Autodesk Inventor part; units mm, degrees
(part 2 of 4)
sketch "스케치25" plane through (0, 5, 0) normal (0, 1, 0) x (1, 0, 0)
  line L0 (49.6203, 83.501) -> (49.6203, 93.501) projected
  arc A0 (51.6203, 95.501) -> (49.6203, 93.501) centre (51.6203, 93.501) ccw projected
  line L1 (51.6203, 95.501) -> (90.0011, 95.501) projected
  arc A1 (92.0011, 93.501) -> (90.0011, 95.501) centre (90.0011, 93.501) ccw projected
  line L2 (92.0011, 93.501) -> (92.0011, 83.501) projected
  arc A2 (90.0011, 81.501) -> (92.0011, 83.501) centre (90.0011, 83.501) ccw projected
  line L3 (90.0011, 81.501) -> (51.6203, 81.501) projected
  arc A3 (49.6203, 83.501) -> (51.6203, 81.501) centre (51.6203, 83.501) ccw projected
  line L4 (127.7787, 126.9669) -> (13, 126.9669) projected
  line L5 (13, 126.9669) -> (-27.1, 106.9169) projected
  line L6 (-27.1, 106.9169) -> (-27.1, -28) projected
  line L7 (-27.1, -28) -> (27.1, -28) projected
  line L8 (27.1, -28) -> (27.1, 45.1435) projected
  arc A4 (28.3615, 47.0022) -> (27.1, 45.1435) centre (29.1, 45.1435) ccw projected
  line L9 (28.3615, 47.0022) -> (126.5171, 85.9998) projected
  arc A5 (126.5171, 85.9998) -> (127.7787, 87.8585) centre (125.7787, 87.8585) ccw projected
  line L10 (127.7787, 126.9669) -> (127.7787, 87.8585) projected
  line L11 (15, 93.501) -> (15, 83.501) projected
  arc A6 (13, 81.501) -> (15, 83.501) centre (13, 83.501) ccw projected
  line L12 (13, 81.501) -> (-13, 81.501) projected
  arc A7 (-15, 83.501) -> (-13, 81.501) centre (-13, 83.501) ccw projected
  line L13 (-15, 83.501) -> (-15, 93.501) projected
  arc A8 (-13, 95.501) -> (-15, 93.501) centre (-13, 93.501) ccw projected
  line L14 (-13, 95.501) -> (13, 95.501) projected
  arc A9 (15, 93.501) -> (13, 95.501) centre (13, 93.501) ccw projected
  circle A10 centre (39.1, 76.501) radius 1.6 projected
  circle A11 centre (49.8107, 76.501) radius 1.6 projected
  circle A12 centre (9.1, 76.501) radius 1.6 projected
  circle A13 centre (-10.9, 76.501) radius 1.6 projected
  circle A14 centre (69.8107, 76.501) radius 1.6 projected
  circle A15 centre (89.8107, 76.501) radius 1.6 projected
  circle A16 centre (12.0104, 4.9749) radius 3.1 projected
  circle A17 centre (4.9749, -12.0104) radius 3.1 projected
  circle A18 centre (-12.0104, -4.9749) radius 3.1 projected
  circle A19 centre (-4.9749, 12.0104) radius 3.1 projected
  circle A20 centre (0, 0) radius 8 projected
  circle A21 centre (-12.0104, 4.9749) radius 3.1 projected
  circle A22 centre (-4.9749, -12.0104) radius 3.1 projected
  circle A23 centre (12.0104, -4.9749) radius 3.1 projected
  circle A24 centre (4.9749, 12.0104) radius 3.1 projected
  circle A25 centre (70.8107, 118.101) radius 1.35 projected
  circle A26 centre (112.9107, 96.101) radius 1.75 projected
  circle A27 centre (58.8107, 106.101) radius 1.35 projected
  circle A28 centre (28.7107, 96.101) radius 1.75 projected
  circle A29 centre (82.8107, 106.101) radius 1.35 projected
  circle A30 centre (112.9107, 116.101) radius 1.75 projected
  circle A31 centre (28.7107, 116.101) radius 1.75 projected
  line L15 (49.6203, 85.501) -> (49.6203, 95.501)
  arc A32 (51.6203, 97.501) -> (49.6203, 95.501) centre (51.6203, 95.501) ccw
  line L16 (51.6203, 97.501) -> (90.0011, 97.501)
  arc A33 (92.0011, 95.501) -> (90.0011, 97.501) centre (90.0011, 95.501) ccw
  line L17 (92.0011, 95.501) -> (92.0011, 85.501)
  arc A34 (90.0011, 83.501) -> (92.0011, 85.501) centre (90.0011, 85.501) ccw
  line L18 (90.0011, 83.501) -> (51.6203, 83.501)
  arc A35 (49.6203, 85.501) -> (51.6203, 83.501) centre (51.6203, 85.501) ccw
  line L19 (127.7787, 128.9669) -> (13, 128.9669)
  line L20 (13, 128.9669) -> (-27.1, 108.9169)
  line L21 (-27.1, 108.9169) -> (-27.1, -26)
  line L22 (-27.1, -26) -> (27.1, -26)
  line L23 (27.1, -26) -> (27.1, 47.1435)
  arc A36 (28.3615, 49.0022) -> (27.1, 47.1435) centre (29.1, 47.1435) ccw
  line L24 (28.3615, 49.0022) -> (126.5171, 87.9998)
  arc A37 (126.5171, 87.9998) -> (127.7787, 89.8585) centre (125.7787, 89.8585) ccw
  line L25 (127.7787, 128.9669) -> (127.7787, 89.8585)
  line L26 (15, 95.501) -> (15, 85.501)
  arc A38 (13, 83.501) -> (15, 85.501) centre (13, 85.501) ccw
  line L27 (13, 83.501) -> (-13, 83.501)
  arc A39 (-15, 85.501) -> (-13, 83.501) centre (-13, 85.501) ccw
  line L28 (-15, 85.501) -> (-15, 95.501)
  arc A40 (-13, 97.501) -> (-15, 95.501) centre (-13, 95.501) ccw
  line L29 (-13, 97.501) -> (13, 97.501)
  arc A41 (15, 95.501) -> (13, 97.501) centre (13, 95.501) ccw
  circle A42 centre (39.1, 78.501) radius 1.6
  circle A43 centre (49.8107, 78.501) radius 1.6
  circle A44 centre (9.1, 78.501) radius 1.6
  circle A45 centre (-10.9, 78.501) radius 1.6
  circle A46 centre (69.8107, 78.501) radius 1.6
  circle A47 centre (89.8107, 78.501) radius 1.6
  circle A48 centre (12.0104, 6.9749) radius 3.1
  circle A49 centre (4.9749, -10.0104) radius 3.1
  circle A50 centre (-12.0104, -2.9749) radius 3.1
  circle A51 centre (-4.9749, 14.0104) radius 3.1
  circle A52 centre (0, 2) radius 8
  circle A53 centre (-12.0104, 6.9749) radius 3.1
  circle A54 centre (-4.9749, -10.0104) radius 3.1
  circle A55 centre (12.0104, -2.9749) radius 3.1
  circle A56 centre (4.9749, 14.0104) radius 3.1
  circle A57 centre (70.8107, 120.101) radius 1.35
  circle A58 centre (112.9107, 98.101) radius 1.75
  circle A59 centre (58.8107, 108.101) radius 1.35
  circle A60 centre (28.7107, 98.101) radius 1.75
  circle A61 centre (82.8107, 108.101) radius 1.35
  circle A62 centre (112.9107, 118.101) radius 1.75
  circle A63 centre (28.7107, 118.101) radius 1.75
  circle A64 centre (70.8107, 118.101) radius 1.35 projected
  line L30 (70.8107, 118.101) -> (70.8107, 120.101)
  point P0 (0, 2)
  dimension "d177" = 2
  constraints: 32 centre point, 32 end point, 20 point on circle, 1 vertical
  measures "d177" distance of L30.start L30.end
extrude "돌출28" add sketch "스케치25" against normal blind 5 contours A25 A57 | A57 L30 A25 | A25 L30 A57 | A26 A58 | A58 A26 | A27 A59 | A59 A27 | A28 A60 | A60 A28 | A29 A61 | A61 A29 | A30 A62 | A62 A30 | A31 A63 | A63 A31 picked at (70.7711, 117.4255) picked at (112.8481, 95.0285) picked at (112.7717, 97.3342) picked at (58.7711, 105.4255) picked at (58.9201, 106.9978) picked at (28.6481, 95.0285) picked at (28.5717, 97.3342) picked at (82.7711, 105.4255) picked at (82.7013, 106.9978) picked at (112.8481, 115.0285) picked at (112.7717, 117.3342) picked at (28.6481, 115.0285) picked at (28.5717, 117.3342)
extrude "돌출29" cut sketch "스케치25" against normal blind 5 contours A57 L30 A25 | A25 A57 | A25 L30 A57 | A58 A26 | A26 A58 | A59 A27 | A27 A59 | A60 A28 | A28 A60 | A61 A29 | A29 A61 | A62 A30 | A30 A62 | A63 A31 | A31 A63 picked at (70.7711, 120.7765) picked at (112.7717, 97.3342) picked at (112.8481, 99.1735) picked at (58.9201, 106.9978) picked at (58.7711, 108.7765) picked at (28.5717, 97.3342) picked at (28.6481, 99.1735) picked at (82.7013, 106.9978) picked at (82.7711, 108.7765) picked at (112.7717, 117.3342) picked at (112.8481, 119.1735) picked at (28.5717, 117.3342) picked at (28.6481, 119.1735)
fillet "모깎기4" radius 2 3 edges at (-27.1, 2.5, -106.9169) (13, 2.5, -126.9669) (127.7787, 2.5, -126.9669)
sketch "스케치26" plane through (0, 5, 0) normal (0, 1, 0) x (1, 0, 0)
  circle A0 centre (4.9749, 12.0104) radius 3.1 projected
  circle A1 centre (12.0104, -4.9749) radius 3.1 projected
  circle A2 centre (-4.9749, -12.0104) radius 3.1 projected
  circle A3 centre (-12.0104, 4.9749) radius 3.1 projected
  circle A4 centre (0, 0) radius 8 projected
  circle A5 centre (-4.9749, 12.0104) radius 3.1 projected
  circle A6 centre (-12.0104, -4.9749) radius 3.1 projected
  circle A7 centre (4.9749, -12.0104) radius 3.1 projected
  circle A8 centre (12.0104, 4.9749) radius 3.1 projected
  circle A9 centre (89.8107, 76.501) radius 1.6 projected
  circle A10 centre (69.8107, 76.501) radius 1.6 projected
  circle A11 centre (-10.9, 76.501) radius 1.6 projected
  circle A12 centre (9.1, 76.501) radius 1.6 projected
  circle A13 centre (49.8107, 76.501) radius 1.6 projected
  circle A14 centre (39.1, 76.501) radius 1.6 projected
  line L0 (15, 93.501) -> (15, 83.501) projected
  arc A15 (13, 81.501) -> (15, 83.501) centre (13, 83.501) ccw projected
  line L1 (13, 81.501) -> (-13, 81.501) projected
  arc A16 (-15, 83.501) -> (-13, 81.501) centre (-13, 83.501) ccw projected
  line L2 (-15, 83.501) -> (-15, 93.501) projected
  arc A17 (-13, 95.501) -> (-15, 93.501) centre (-13, 93.501) ccw projected
  line L3 (-13, 95.501) -> (13, 95.501) projected
  arc A18 (15, 93.501) -> (13, 95.501) centre (13, 93.501) ccw projected
  arc A19 (127.7787, 124.9669) -> (125.7787, 126.9669) centre (125.7787, 124.9669) ccw projected
  line L4 (125.7787, 126.9669) -> (13.4721, 126.9669) projected
  arc A20 (13.4721, 126.9669) -> (12.5777, 126.7557) centre (13.4721, 124.9669) ccw projected
  line L5 (12.5777, 126.7557) -> (-25.9944, 107.4697) projected
  arc A21 (-25.9944, 107.4697) -> (-27.1, 105.6808) centre (-25.1, 105.6808) ccw projected
  line L6 (-27.1, 105.6808) -> (-27.1, -28) projected
  line L7 (-27.1, -28) -> (27.1, -28) projected
  line L8 (27.1, -28) -> (27.1, 45.1435) projected
  arc A22 (28.3615, 47.0022) -> (27.1, 45.1435) centre (29.1, 45.1435) ccw projected
  line L9 (28.3615, 47.0022) -> (126.5171, 85.9998) projected
  arc A23 (126.5171, 85.9998) -> (127.7787, 87.8585) centre (125.7787, 87.8585) ccw projected
  line L10 (127.7787, 124.9669) -> (127.7787, 87.8585) projected
  line L11 (49.6203, 83.501) -> (49.6203, 93.501) projected
  arc A24 (51.6203, 95.501) -> (49.6203, 93.501) centre (51.6203, 93.501) ccw projected
  line L12 (51.6203, 95.501) -> (90.0011, 95.501) projected
  arc A25 (92.0011, 93.501) -> (90.0011, 95.501) centre (90.0011, 93.501) ccw projected
  line L13 (92.0011, 93.501) -> (92.0011, 83.501) projected
  arc A26 (90.0011, 81.501) -> (92.0011, 83.501) centre (90.0011, 83.501) ccw projected
  line L14 (90.0011, 81.501) -> (51.6203, 81.501) projected
  arc A27 (49.6203, 83.501) -> (51.6203, 81.501) centre (51.6203, 83.501) ccw projected
  circle A28 centre (28.7107, 98.101) radius 1.75 projected
  circle A29 centre (82.8107, 108.101) radius 1.35 projected
  circle A30 centre (112.9107, 118.101) radius 1.75 projected
  circle A31 centre (28.7107, 118.101) radius 1.75 projected
  circle A32 centre (70.8107, 120.101) radius 1.35 projected
  circle A33 centre (112.9107, 98.101) radius 1.75 projected
  circle A34 centre (58.8107, 108.101) radius 1.35 projected
  line L15 (-27.1, 105.6808) -> (-27.1, -28) projected
  line L16 (-27.1, 0) -> (27.1, 0)
  line L17 (27.1, -28) -> (27.1, 45.1435) projected
  point P0 (27.1, 0)
  constraints: 2 end point, 2 point on line
extrude "돌출30" cut sketch "스케치26" against normal blind 10 contours A1 | A2 | L16 L8 L7 L6 A4 | A4 L16 | A6 | A7 picked at (-2.3612, -1.2393)
sketch "스케치27" plane through (0, 5, 0) normal (0, 1, 0) x (1, 0, 0)
  circle A0 centre (58.8107, 108.101) radius 1.35 projected
  circle A1 centre (112.9107, 98.101) radius 1.75 projected
  circle A2 centre (70.8107, 120.101) radius 1.35 projected
  circle A3 centre (28.7107, 118.101) radius 1.75 projected
  circle A4 centre (112.9107, 118.101) radius 1.75 projected
  circle A5 centre (82.8107, 108.101) radius 1.35 projected
  circle A6 centre (28.7107, 98.101) radius 1.75 projected
  line L0 (49.6203, 83.501) -> (49.6203, 93.501) projected
  arc A7 (51.6203, 95.501) -> (49.6203, 93.501) centre (51.6203, 93.501) ccw projected
  line L1 (51.6203, 95.501) -> (90.0011, 95.501) projected
  arc A8 (92.0011, 93.501) -> (90.0011, 95.501) centre (90.0011, 93.501) ccw projected
  line L2 (92.0011, 93.501) -> (92.0011, 83.501) projected
  arc A9 (90.0011, 81.501) -> (92.0011, 83.501) centre (90.0011, 83.501) ccw projected
  line L3 (90.0011, 81.501) -> (51.6203, 81.501) projected
  arc A10 (49.6203, 83.501) -> (51.6203, 81.501) centre (51.6203, 83.501) ccw projected
  line L4 (-27.1, 0) -> (-8, 0) projected
  arc A11 (8, 0) -> (-8, 0) centre (0, 0) ccw projected
  line L5 (8, 0) -> (27.1, 0) projected
  line L6 (27.1, 0) -> (27.1, 45.1435) projected
  arc A12 (28.3615, 47.0022) -> (27.1, 45.1435) centre (29.1, 45.1435) ccw projected
  line L7 (28.3615, 47.0022) -> (126.5171, 85.9998) projected
  arc A13 (126.5171, 85.9998) -> (127.7787, 87.8585) centre (125.7787, 87.8585) ccw projected
  line L8 (127.7787, 124.9669) -> (127.7787, 87.8585) projected
  arc A14 (127.7787, 124.9669) -> (125.7787, 126.9669) centre (125.7787, 124.9669) ccw projected
  line L9 (125.7787, 126.9669) -> (13.4721, 126.9669) projected
  arc A15 (13.4721, 126.9669) -> (12.5777, 126.7557) centre (13.4721, 124.9669) ccw projected
  line L10 (12.5777, 126.7557) -> (-25.9944, 107.4697) projected
  arc A16 (-25.9944, 107.4697) -> (-27.1, 105.6808) centre (-25.1, 105.6808) ccw projected
  line L11 (-27.1, 105.6808) -> (-27.1, 0) projected
  line L12 (15, 93.501) -> (15, 83.501) projected
  arc A17 (13, 81.501) -> (15, 83.501) centre (13, 83.501) ccw projected
  line L13 (13, 81.501) -> (-13, 81.501) projected
  arc A18 (-15, 83.501) -> (-13, 81.501) centre (-13, 83.501) ccw projected
  line L14 (-15, 83.501) -> (-15, 93.501) projected
  arc A19 (-13, 95.501) -> (-15, 93.501) centre (-13, 93.501) ccw projected
  line L15 (-13, 95.501) -> (13, 95.501) projected
  arc A20 (15, 93.501) -> (13, 95.501) centre (13, 93.501) ccw projected
  circle A21 centre (39.1, 76.501) radius 1.6 projected
  circle A22 centre (49.8107, 76.501) radius 1.6 projected
  circle A23 centre (9.1, 76.501) radius 1.6 projected
  circle A24 centre (-10.9, 76.501) radius 1.6 projected
  circle A25 centre (69.8107, 76.501) radius 1.6 projected
  circle A26 centre (89.8107, 76.501) radius 1.6 projected
  circle A27 centre (12.0104, 4.9749) radius 3.1 projected
  circle A28 centre (-4.9749, 12.0104) radius 3.1 projected
  circle A29 centre (-12.0104, 4.9749) radius 3.1 projected
  circle A30 centre (4.9749, 12.0104) radius 3.1 projected
  circle A31 centre (12.0104, 4.9749) radius 1.6 projected
  circle A32 centre (4.9749, 12.0104) radius 1.6 projected
  circle A33 centre (-4.9749, 12.0104) radius 1.6 projected
  circle A34 centre (-12.0104, 4.9749) radius 1.6 projected
  line L16 (27.1, 0) -> (27.1, 45.1435) projected
  line L17 (-27.1, 0) -> (-27.1, 105.6808) projected
  line L18 (27.1, 0) -> (-27.1, 0)
  circle A35 centre (58.8107, -108.101) radius 1.35
  circle A36 centre (112.9107, -98.101) radius 1.75
  circle A37 centre (70.8107, -120.101) radius 1.35
  circle A38 centre (28.7107, -118.101) radius 1.75
  circle A39 centre (112.9107, -118.101) radius 1.75
  circle A40 centre (82.8107, -108.101) radius 1.35
  circle A41 centre (28.7107, -98.101) radius 1.75
  line L19 (49.6203, -83.501) -> (49.6203, -93.501)
  arc A42 (49.6203, -93.501) -> (51.6203, -95.501) centre (51.6203, -93.501) ccw
  line L20 (51.6203, -95.501) -> (90.0011, -95.501)
  arc A43 (90.0011, -95.501) -> (92.0011, -93.501) centre (90.0011, -93.501) ccw
  line L21 (92.0011, -93.501) -> (92.0011, -83.501)
  arc A44 (92.0011, -83.501) -> (90.0011, -81.501) centre (90.0011, -83.501) ccw
  line L22 (90.0011, -81.501) -> (51.6203, -81.501)
  arc A45 (51.6203, -81.501) -> (49.6203, -83.501) centre (51.6203, -83.501) ccw
  arc A46 (-8, 0) -> (8, 0) centre (0, 0) ccw
  line L23 (27.1, 0) -> (27.1, -45.1435)
  arc A47 (27.1, -45.1435) -> (28.3615, -47.0022) centre (29.1, -45.1435) ccw
  line L24 (28.3615, -47.0022) -> (126.5171, -85.9998)
  arc A48 (127.7787, -87.8585) -> (126.5171, -85.9998) centre (125.7787, -87.8585) ccw
  line L25 (127.7787, -124.9669) -> (127.7787, -87.8585)
  arc A49 (125.7787, -126.9669) -> (127.7787, -124.9669) centre (125.7787, -124.9669) ccw
  line L26 (125.7787, -126.9669) -> (13.4721, -126.9669)
  arc A50 (12.5777, -126.7557) -> (13.4721, -126.9669) centre (13.4721, -124.9669) ccw
  line L27 (12.5777, -126.7557) -> (-25.9944, -107.4697)
  arc A51 (-27.1, -105.6808) -> (-25.9944, -107.4697) centre (-25.1, -105.6808) ccw
  line L28 (-27.1, -105.6808) -> (-27.1, 0)
  line L29 (15, -93.501) -> (15, -83.501)
  arc A52 (15, -83.501) -> (13, -81.501) centre (13, -83.501) ccw
  line L30 (13, -81.501) -> (-13, -81.501)
  arc A53 (-13, -81.501) -> (-15, -83.501) centre (-13, -83.501) ccw
  line L31 (-15, -83.501) -> (-15, -93.501)
  arc A54 (-15, -93.501) -> (-13, -95.501) centre (-13, -93.501) ccw
  line L32 (-13, -95.501) -> (13, -95.501)
  arc A55 (13, -95.501) -> (15, -93.501) centre (13, -93.501) ccw
  circle A56 centre (39.1, -76.501) radius 1.6
  circle A57 centre (49.8107, -76.501) radius 1.6
  circle A58 centre (9.1, -76.501) radius 1.6
  circle A59 centre (-10.9, -76.501) radius 1.6
  circle A60 centre (69.8107, -76.501) radius 1.6
  circle A61 centre (89.8107, -76.501) radius 1.6
  circle A62 centre (12.0104, -4.9749) radius 3.1
  circle A63 centre (-4.9749, -12.0104) radius 3.1
  circle A64 centre (-12.0104, -4.9749) radius 3.1
  circle A65 centre (4.9749, -12.0104) radius 3.1
  circle A66 centre (12.0104, -4.9749) radius 1.6
  circle A67 centre (4.9749, -12.0104) radius 1.6
  circle A68 centre (-4.9749, -12.0104) radius 1.6
  circle A69 centre (-12.0104, -4.9749) radius 1.6
  line L33 (27.1, 0) -> (27.1, -45.1435)
  line L34 (-27.1, 0) -> (-27.1, -105.6808)
  constraints: 60 symmetric about line, 35 centre point, 34 end point, 28 point on circle, 1 perpendicular, 35 other
extrude "돌출31" add sketch "스케치27" against normal blind 5 contours L4 A46 L5 L23 A47 L24 A48 L25 A49 L26 A50 L27 A51 L28
sketch "스케치28" plane through (0, 5, 0) normal (0, 1, 0) x (1, 0, 0)
  line L0 (27.1, -45.1435) -> (27.1, 45.1435) projected
  arc A0 (28.3615, 47.0022) -> (27.1, 45.1435) centre (29.1, 45.1435) ccw projected
  line L1 (28.3615, 47.0022) -> (126.5171, 85.9998) projected
  arc A1 (126.5171, 85.9998) -> (127.7787, 87.8585) centre (125.7787, 87.8585) ccw projected
  line L2 (127.7787, 124.9669) -> (127.7787, 87.8585) projected
  arc A2 (127.7787, 124.9669) -> (125.7787, 126.9669) centre (125.7787, 124.9669) ccw projected
  line L3 (125.7787, 126.9669) -> (13.4721, 126.9669) projected
  arc A3 (13.4721, 126.9669) -> (12.5777, 126.7557) centre (13.4721, 124.9669) ccw projected
  line L4 (12.5777, 126.7557) -> (-25.9944, 107.4697) projected
  arc A4 (-25.9944, 107.4697) -> (-27.1, 105.6808) centre (-25.1, 105.6808) ccw projected
  line L5 (-27.1, 105.6808) -> (-27.1, -105.6808) projected
  arc A5 (-27.1, -105.6808) -> (-25.9944, -107.4697) centre (-25.1, -105.6808) ccw projected
  line L6 (-25.9944, -107.4697) -> (12.5777, -126.7557) projected
  arc A6 (12.5777, -126.7557) -> (13.4721, -126.9669) centre (13.4721, -124.9669) ccw projected
  line L7 (13.4721, -126.9669) -> (125.7787, -126.9669) projected
  arc A7 (125.7787, -126.9669) -> (127.7787, -124.9669) centre (125.7787, -124.9669) ccw projected
  line L8 (127.7787, -124.9669) -> (127.7787, -87.8585) projected
  arc A8 (127.7787, -87.8585) -> (126.5171, -85.9998) centre (125.7787, -87.8585) ccw projected
  line L9 (126.5171, -85.9998) -> (28.3615, -47.0022) projected
  arc A9 (27.1, -45.1435) -> (28.3615, -47.0022) centre (29.1, -45.1435) ccw projected
  arc A10 (15, -83.501) -> (13, -81.501) centre (13, -83.501) ccw projected
  line L10 (15, -83.501) -> (15, -93.501) projected
  arc A11 (13, -95.501) -> (15, -93.501) centre (13, -93.501) ccw projected
  line L11 (13, -95.501) -> (-13, -95.501) projected
  arc A12 (-15, -93.501) -> (-13, -95.501) centre (-13, -93.501) ccw projected
  line L12 (-15, -93.501) -> (-15, -83.501) projected
  arc A13 (-13, -81.501) -> (-15, -83.501) centre (-13, -83.501) ccw projected
  line L13 (-13, -81.501) -> (13, -81.501) projected
  line L14 (49.6203, -93.501) -> (49.6203, -83.501) projected
  arc A14 (51.6203, -81.501) -> (49.6203, -83.501) centre (51.6203, -83.501) ccw projected
  line L15 (51.6203, -81.501) -> (90.0011, -81.501) projected
  arc A15 (92.0011, -83.501) -> (90.0011, -81.501) centre (90.0011, -83.501) ccw projected
  line L16 (92.0011, -83.501) -> (92.0011, -93.501) projected
  arc A16 (90.0011, -95.501) -> (92.0011, -93.501) centre (90.0011, -93.501) ccw projected
  line L17 (90.0011, -95.501) -> (51.6203, -95.501) projected
  arc A17 (49.6203, -93.501) -> (51.6203, -95.501) centre (51.6203, -93.501) ccw projected
  circle A18 centre (49.8107, -76.501) radius 1.6 projected
  circle A19 centre (39.1, -76.501) radius 1.6 projected
  circle A20 centre (69.8107, -76.501) radius 1.6 projected
  circle A21 centre (89.8107, -76.501) radius 1.6 projected
  circle A22 centre (-4.9749, -12.0104) radius 3.1 projected
  circle A23 centre (4.9749, -12.0104) radius 3.1 projected
  circle A24 centre (-12.0104, -4.9749) radius 3.1 projected
  circle A25 centre (12.0104, -4.9749) radius 3.1 projected
  circle A26 centre (9.1, -76.501) radius 1.6 projected
  circle A27 centre (112.9107, -98.101) radius 1.75 projected
  circle A28 centre (82.8107, -108.101) radius 1.35 projected
  circle A29 centre (58.8107, -108.101) radius 1.35 projected
  circle A30 centre (28.7107, -118.101) radius 1.75 projected
  circle A31 centre (28.7107, -98.101) radius 1.75 projected
  circle A32 centre (70.8107, -120.101) radius 1.35 projected
  circle A33 centre (112.9107, -118.101) radius 1.75 projected
  circle A34 centre (-10.9, -76.501) radius 1.6 projected
  circle A35 centre (58.8107, 108.101) radius 1.35 projected
  circle A36 centre (112.9107, 98.101) radius 1.75 projected
  circle A37 centre (70.8107, 120.101) radius 1.35 projected
  circle A38 centre (28.7107, 118.101) radius 1.75 projected
  circle A39 centre (112.9107, 118.101) radius 1.75 projected
  circle A40 centre (82.8107, 108.101) radius 1.35 projected
  circle A41 centre (28.7107, 98.101) radius 1.75 projected
  line L18 (49.6203, 83.501) -> (49.6203, 93.501) projected
  arc A42 (51.6203, 95.501) -> (49.6203, 93.501) centre (51.6203, 93.501) ccw projected
  line L19 (51.6203, 95.501) -> (90.0011, 95.501) projected
  arc A43 (92.0011, 93.501) -> (90.0011, 95.501) centre (90.0011, 93.501) ccw projected
  line L20 (92.0011, 93.501) -> (92.0011, 83.501) projected
  arc A44 (90.0011, 81.501) -> (92.0011, 83.501) centre (90.0011, 83.501) ccw projected
  line L21 (90.0011, 81.501) -> (51.6203, 81.501) projected
  arc A45 (49.6203, 83.501) -> (51.6203, 81.501) centre (51.6203, 83.501) ccw projected
  circle A46 centre (0, 0) radius 8 projected
  line L22 (15, 93.501) -> (15, 83.501) projected
  arc A47 (13, 81.501) -> (15, 83.501) centre (13, 83.501) ccw projected
  line L23 (13, 81.501) -> (-13, 81.501) projected
  arc A48 (-15, 83.501) -> (-13, 81.501) centre (-13, 83.501) ccw projected
  line L24 (-15, 83.501) -> (-15, 93.501) projected
  arc A49 (-13, 95.501) -> (-15, 93.501) centre (-13, 93.501) ccw projected
  line L25 (-13, 95.501) -> (13, 95.501) projected
  arc A50 (15, 93.501) -> (13, 95.501) centre (13, 93.501) ccw projected
  circle A51 centre (39.1, 76.501) radius 1.6 projected
  circle A52 centre (49.8107, 76.501) radius 1.6 projected
  circle A53 centre (9.1, 76.501) radius 1.6 projected
  circle A54 centre (-10.9, 76.501) radius 1.6 projected
  circle A55 centre (69.8107, 76.501) radius 1.6 projected
  circle A56 centre (89.8107, 76.501) radius 1.6 projected
  circle A57 centre (12.0104, 4.9749) radius 3.1 projected
  circle A58 centre (-4.9749, 12.0104) radius 3.1 projected
  circle A59 centre (-12.0104, 4.9749) radius 3.1 projected
  circle A60 centre (4.9749, 12.0104) radius 3.1 projected
  circle A61 centre (28.7107, 118.101) radius 1.75 projected
  line L26 (28.7107, 98.101) -> (28.7107, 118.101)
  circle A62 centre (35.7787, 108.101) radius 1.75
  circle A63 centre (15.7787, 108.101) radius 1.85
  line L27 (27.1, -45.1435) -> (27.1, 45.1435) projected
  line L28 (27.1, 0) -> (-27.1, 0)
  line L29 (-27.1, -105.6808) -> (-27.1, 105.6808) projected
  line L30 (125.7787, -126.9669) -> (13.4721, -126.9669)
  circle A64 centre (28.7107, -118.101) radius 1.75
  circle A65 centre (28.7107, -98.101) radius 1.75
  circle A66 centre (28.7107, -118.101) radius 1.75
  line L31 (28.7107, -98.101) -> (28.7107, -118.101)
  circle A67 centre (25.7787, -108.5308) radius 10.0092
  circle A68 centre (35.7787, -108.101) radius 1.75
  circle A69 centre (15.7787, -108.101) radius 1.85
  circle A70 centre (112.9107, 118.101) radius 1.75
  circle A71 centre (109.9787, 98.101) radius 1.75
  circle A72 centre (109.9787, 118.101) radius 1.75
  line L32 (109.9787, 98.101) -> (109.9787, 118.101)
  circle A73 centre (119.9787, 108.101) radius 1.75
  circle A74 centre (99.9787, 108.101) radius 1.85
  circle A75 centre (112.9107, 118.101) radius 1.75 projected
  line L33 (112.9107, 118.101) -> (112.9107, 98.101)
  circle A76 centre (112.9107, -98.101) radius 1.75
  circle A77 centre (112.9107, -118.101) radius 1.75
  circle A78 centre (112.9107, -118.101) radius 1.75
  circle A79 centre (119.9787, -108.101) radius 1.75
  circle A80 centre (109.9787, -98.101) radius 1.75
  line L34 (109.9787, -98.101) -> (109.9787, -118.101)
  circle A81 centre (109.9787, -118.101) radius 1.75
  circle A82 centre (109.9787, -108.101) radius 10
  circle A83 centre (99.9787, -108.101) radius 1.85
  circle A84 centre (112.9107, -118.101) radius 1.75
  line L35 (112.9107, -118.101) -> (112.9107, -98.101)
  point P0 (112.9107, 108.101)
  point P1 (112.9107, -108.101)
  dimension "d187" = 3.5
  dimension "d188" = 3.7
  dimension "d191" = 3.5
  dimension "d192" = 3.7
  dimension "d196" = 20
  dimension "d197" = 18.8659
  dimension "d198" = 7.8
  dimension "d199" = 64.2
  dimension "d200" = 20
  constraints: 22 centre point, 14 end point, 14 symmetric about line, 6 point on circle, 3 midpoint, 3 vertical, 16 other
  measures "d187" diameter of A62
  measures "d188" diameter of A63
  measures "d191" diameter of A73
  measures "d192" diameter of A74
  measures "d196" distance of A74.centre A73.centre
  measures "d197" distance from line of L3 A73.centre
  measures "d198" distance from line of L2 A73.centre
  measures "d199" distance of A62.centre A74.centre
  measures "d200" distance of A63.centre A62.centre
extrude "돌출32" cut sketch "스케치28" against normal blind 5 contours A82 A79 | A79 A82 | A83 A82 | A82 A83 | A68 A67 | A67 A68 | A69 A67 | A67 A69 | A62 | A63 | A73 | A74
sketch "스케치29" plane through (0, 5, 0) normal (0, 1, 0) x (1, 0, 0)
  circle A0 centre (99.9787, 108.101) radius 1.85 projected
  circle A1 centre (15.7787, -108.101) radius 1.85 projected
  circle A2 centre (35.7787, 108.101) radius 1.75 projected
  circle A3 centre (119.9787, -108.101) radius 1.75 projected
  circle A4 centre (119.9787, 108.101) radius 1.75 projected
  circle A5 centre (35.7787, -108.101) radius 1.75 projected
  circle A6 centre (15.7787, 108.101) radius 1.85 projected
  circle A7 centre (99.9787, -108.101) radius 1.85 projected
  line L0 (27.1, -45.1435) -> (27.1, 45.1435) projected
  arc A8 (28.3615, 47.0022) -> (27.1, 45.1435) centre (29.1, 45.1435) ccw projected
  line L1 (28.3615, 47.0022) -> (126.5171, 85.9998) projected
  arc A9 (126.5171, 85.9998) -> (127.7787, 87.8585) centre (125.7787, 87.8585) ccw projected
  line L2 (127.7787, 124.9669) -> (127.7787, 87.8585) projected
  arc A10 (127.7787, 124.9669) -> (125.7787, 126.9669) centre (125.7787, 124.9669) ccw projected
  line L3 (125.7787, 126.9669) -> (13.4721, 126.9669) projected
  arc A11 (13.4721, 126.9669) -> (12.5777, 126.7557) centre (13.4721, 124.9669) ccw projected
  line L4 (12.5777, 126.7557) -> (-25.9944, 107.4697) projected
  arc A12 (-25.9944, 107.4697) -> (-27.1, 105.6808) centre (-25.1, 105.6808) ccw projected
  line L5 (-27.1, 105.6808) -> (-27.1, -105.6808) projected
  arc A13 (-27.1, -105.6808) -> (-25.9944, -107.4697) centre (-25.1, -105.6808) ccw projected
  line L6 (-25.9944, -107.4697) -> (12.5777, -126.7557) projected
  arc A14 (12.5777, -126.7557) -> (13.4721, -126.9669) centre (13.4721, -124.9669) ccw projected
  line L7 (13.4721, -126.9669) -> (125.7787, -126.9669) projected
  arc A15 (125.7787, -126.9669) -> (127.7787, -124.9669) centre (125.7787, -124.9669) ccw projected
  line L8 (127.7787, -124.9669) -> (127.7787, -87.8585) projected
  arc A16 (127.7787, -87.8585) -> (126.5171, -85.9998) centre (125.7787, -87.8585) ccw projected
  line L9 (126.5171, -85.9998) -> (28.3615, -47.0022) projected
  arc A17 (27.1, -45.1435) -> (28.3615, -47.0022) centre (29.1, -45.1435) ccw projected
  arc A18 (15, -83.501) -> (13, -81.501) centre (13, -83.501) ccw projected
  line L10 (15, -83.501) -> (15, -93.501) projected
  arc A19 (13, -95.501) -> (15, -93.501) centre (13, -93.501) ccw projected
  line L11 (13, -95.501) -> (-13, -95.501) projected
  arc A20 (-15, -93.501) -> (-13, -95.501) centre (-13, -93.501) ccw projected
  line L12 (-15, -93.501) -> (-15, -83.501) projected
  arc A21 (-13, -81.501) -> (-15, -83.501) centre (-13, -83.501) ccw projected
  line L13 (-13, -81.501) -> (13, -81.501) projected
  line L14 (49.6203, -93.501) -> (49.6203, -83.501) projected
  arc A22 (51.6203, -81.501) -> (49.6203, -83.501) centre (51.6203, -83.501) ccw projected
  line L15 (51.6203, -81.501) -> (90.0011, -81.501) projected
  arc A23 (92.0011, -83.501) -> (90.0011, -81.501) centre (90.0011, -83.501) ccw projected
  line L16 (92.0011, -83.501) -> (92.0011, -93.501) projected
  arc A24 (90.0011, -95.501) -> (92.0011, -93.501) centre (90.0011, -93.501) ccw projected
  line L17 (90.0011, -95.501) -> (51.6203, -95.501) projected
  arc A25 (49.6203, -93.501) -> (51.6203, -95.501) centre (51.6203, -93.501) ccw projected
  circle A26 centre (49.8107, -76.501) radius 1.6 projected
  circle A27 centre (39.1, -76.501) radius 1.6 projected
  circle A28 centre (69.8107, -76.501) radius 1.6 projected
  circle A29 centre (89.8107, -76.501) radius 1.6 projected
  circle A30 centre (-4.9749, -12.0104) radius 3.1 projected
  circle A31 centre (4.9749, -12.0104) radius 3.1 projected
  circle A32 centre (-12.0104, -4.9749) radius 3.1 projected
  circle A33 centre (12.0104, -4.9749) radius 3.1 projected
  circle A34 centre (9.1, -76.501) radius 1.6 projected
  circle A35 centre (112.9107, -98.101) radius 1.75 projected
  circle A36 centre (82.8107, -108.101) radius 1.35 projected
  circle A37 centre (58.8107, -108.101) radius 1.35 projected
  circle A38 centre (28.7107, -118.101) radius 1.75 projected
  circle A39 centre (28.7107, -98.101) radius 1.75 projected
  circle A40 centre (70.8107, -120.101) radius 1.35 projected
  circle A41 centre (112.9107, -118.101) radius 1.75 projected
  circle A42 centre (-10.9, -76.501) radius 1.6 projected
  circle A43 centre (58.8107, 108.101) radius 1.35 projected
  circle A44 centre (112.9107, 98.101) radius 1.75 projected
  circle A45 centre (70.8107, 120.101) radius 1.35 projected
  circle A46 centre (28.7107, 118.101) radius 1.75 projected
  circle A47 centre (112.9107, 118.101) radius 1.75 projected
  circle A48 centre (82.8107, 108.101) radius 1.35 projected
  circle A49 centre (28.7107, 98.101) radius 1.75 projected
  line L18 (49.6203, 83.501) -> (49.6203, 93.501) projected
  arc A50 (51.6203, 95.501) -> (49.6203, 93.501) centre (51.6203, 93.501) ccw projected
  line L19 (51.6203, 95.501) -> (90.0011, 95.501) projected
  arc A51 (92.0011, 93.501) -> (90.0011, 95.501) centre (90.0011, 93.501) ccw projected
  line L20 (92.0011, 93.501) -> (92.0011, 83.501) projected
  arc A52 (90.0011, 81.501) -> (92.0011, 83.501) centre (90.0011, 83.501) ccw projected
  line L21 (90.0011, 81.501) -> (51.6203, 81.501) projected
  arc A53 (49.6203, 83.501) -> (51.6203, 81.501) centre (51.6203, 83.501) ccw projected
  circle A54 centre (0, 0) radius 8 projected
  line L22 (15, 93.501) -> (15, 83.501) projected
  arc A55 (13, 81.501) -> (15, 83.501) centre (13, 83.501) ccw projected
  line L23 (13, 81.501) -> (-13, 81.501) projected
  arc A56 (-15, 83.501) -> (-13, 81.501) centre (-13, 83.501) ccw projected
  line L24 (-15, 83.501) -> (-15, 93.501) projected
  arc A57 (-13, 95.501) -> (-15, 93.501) centre (-13, 93.501) ccw projected
  line L25 (-13, 95.501) -> (13, 95.501) projected
  arc A58 (15, 93.501) -> (13, 95.501) centre (13, 93.501) ccw projected
  circle A59 centre (39.1, 76.501) radius 1.6 projected
  circle A60 centre (49.8107, 76.501) radius 1.6 projected
  circle A61 centre (9.1, 76.501) radius 1.6 projected
  circle A62 centre (-10.9, 76.501) radius 1.6 projected
  circle A63 centre (69.8107, 76.501) radius 1.6 projected
  circle A64 centre (89.8107, 76.501) radius 1.6 projected
  circle A65 centre (12.0104, 4.9749) radius 3.1 projected
  circle A66 centre (-4.9749, 12.0104) radius 3.1 projected
  circle A67 centre (-12.0104, 4.9749) radius 3.1 projected
  circle A68 centre (4.9749, 12.0104) radius 3.1 projected
  arc A69 (28.3615, 47.0022) -> (27.1, 45.1435) centre (29.1, 45.1435) ccw projected
  line L26 (27.1, 45.1435) -> (27.1, 33.1435)
  line L27 (27.1, 33.1435) -> (127.7787, 73.1435)
  line L28 (28.3615, 47.0022) -> (126.5171, 85.9998) projected
  arc A70 (126.5171, 85.9998) -> (127.7787, 87.8585) centre (125.7787, 87.8585) ccw projected
  line L29 (127.7787, 87.8585) -> (127.7787, 73.1435)
  line L30 (27.1, -45.1435) -> (27.1, 45.1435) projected
  line L31 (27.1, 0) -> (-27.1, 0)
  line L32 (-27.1, 105.6808) -> (-27.1, -105.6808) projected
  line L33 (27.1, -33.1435) -> (127.7787, -73.1435)
  line L34 (127.7787, -87.8585) -> (127.7787, -73.1435)
  arc A71 (-25.9944, 107.4697) -> (-27.1, 105.6808) centre (-25.1, 105.6808) ccw projected
  line L35 (-27.1, 105.6808) -> (-27.1, 132.9669)
  arc A72 (127.7787, 124.9669) -> (125.7787, 126.9669) centre (125.7787, 124.9669) ccw projected
  line L36 (127.7787, 124.9669) -> (127.7787, 132.9669)
  line L37 (127.7787, 132.9669) -> (-27.1, 132.9669)
  line L38 (-27.1, -105.6808) -> (-27.1, -132.9669)
  line L39 (127.7787, -124.9669) -> (127.7787, -132.9669)
  line L40 (127.7787, -132.9669) -> (-27.1, -132.9669)
  point P0 (27.1, -33.1435)
  dimension "d201" = 12
  dimension "d204" = 8
  constraints: 24 end point, 4 symmetric about line, 3 tangent, 3 vertical, 2 midpoint, 1 parallel, 1 perpendicular, 1 point on line
  measures "d201" distance of L0.end L26.end
  measures "d204" distance of L2.start L36.end
extrude "돌출33" add sketch "스케치29" against normal blind 5 contours L0 L33 L34 A16 L9 A17 | L0 A8 L1 A9 L29 L27 | L39 L40 L38 A13 L6 A14 L7 A15 | A10 L3 A11 L4 A12 L35 L37 L36
fillet "모깎기5" radius 12 8 edges at (127.7787, 2.5, -132.9669) (127.7787, 2.5, -73.1435) (27.1, 2.5, -33.1435) (27.1, 2.5, 33.1435) (127.7787, 2.5, 73.1435) (127.7787, 2.5, 132.9669) (-27.1, 2.5, 132.9669) (-27.1, 2.5, -132.9669)
sketch "스케치30" plane through (0, 5, 0) normal (0, 1, 0) x (1, 0, 0)
  circle A0 centre (99.9787, 108.101) radius 1.85 projected
  circle A1 centre (15.7787, -108.101) radius 1.85 projected
  circle A2 centre (35.7787, 108.101) radius 1.75 projected
  circle A3 centre (119.9787, -108.101) radius 1.75 projected
  circle A4 centre (119.9787, 108.101) radius 1.75 projected
  circle A5 centre (35.7787, -108.101) radius 1.75 projected
  circle A6 centre (15.7787, 108.101) radius 1.85 projected
  circle A7 centre (99.9787, -108.101) radius 1.85 projected
  arc A8 (-15.1, 132.9669) -> (-27.1, 120.9669) centre (-15.1, 120.9669) ccw projected
  line L0 (-27.1, 120.9669) -> (-27.1, -120.9669) projected
  arc A9 (-27.1, -120.9669) -> (-15.1, -132.9669) centre (-15.1, -120.9669) ccw projected
  line L1 (-15.1, -132.9669) -> (115.7787, -132.9669) projected
  arc A10 (115.7787, -132.9669) -> (127.7787, -120.9669) centre (115.7787, -120.9669) ccw projected
  line L2 (127.7787, -120.9669) -> (127.7787, -81.2883) projected
  arc A11 (127.7787, -81.2883) -> (120.2094, -70.1362) centre (115.7787, -81.2883) ccw projected
  line L3 (120.2094, -70.1362) -> (34.6692, -36.1508) projected
  arc A12 (27.1, -24.9988) -> (34.6692, -36.1508) centre (39.1, -24.9988) ccw projected
  line L4 (27.1, -24.9988) -> (27.1, 24.9988) projected
  arc A13 (34.6692, 36.1508) -> (27.1, 24.9988) centre (39.1, 24.9988) ccw projected
  line L5 (34.6692, 36.1508) -> (120.2094, 70.1362) projected
  arc A14 (120.2094, 70.1362) -> (127.7787, 81.2883) centre (115.7787, 81.2883) ccw projected
  line L6 (127.7787, 81.2883) -> (127.7787, 120.9669) projected
  arc A15 (127.7787, 120.9669) -> (115.7787, 132.9669) centre (115.7787, 120.9669) ccw projected
  line L7 (115.7787, 132.9669) -> (-15.1, 132.9669) projected
  arc A16 (15, -83.501) -> (13, -81.501) centre (13, -83.501) ccw projected
  line L8 (15, -83.501) -> (15, -93.501) projected
  arc A17 (13, -95.501) -> (15, -93.501) centre (13, -93.501) ccw projected
  line L9 (13, -95.501) -> (-13, -95.501) projected
  arc A18 (-15, -93.501) -> (-13, -95.501) centre (-13, -93.501) ccw projected
  line L10 (-15, -93.501) -> (-15, -83.501) projected
  arc A19 (-13, -81.501) -> (-15, -83.501) centre (-13, -83.501) ccw projected
  line L11 (-13, -81.501) -> (13, -81.501) projected
  line L12 (49.6203, -93.501) -> (49.6203, -83.501) projected
  arc A20 (51.6203, -81.501) -> (49.6203, -83.501) centre (51.6203, -83.501) ccw projected
  line L13 (51.6203, -81.501) -> (90.0011, -81.501) projected
  arc A21 (92.0011, -83.501) -> (90.0011, -81.501) centre (90.0011, -83.501) ccw projected
  line L14 (92.0011, -83.501) -> (92.0011, -93.501) projected
  arc A22 (90.0011, -95.501) -> (92.0011, -93.501) centre (90.0011, -93.501) ccw projected
  line L15 (90.0011, -95.501) -> (51.6203, -95.501) projected
  arc A23 (49.6203, -93.501) -> (51.6203, -95.501) centre (51.6203, -93.501) ccw projected
  circle A24 centre (49.8107, -76.501) radius 1.6 projected
  circle A25 centre (39.1, -76.501) radius 1.6 projected
  circle A26 centre (69.8107, -76.501) radius 1.6 projected
  circle A27 centre (89.8107, -76.501) radius 1.6 projected
  circle A28 centre (-4.9749, -12.0104) radius 3.1 projected
  circle A29 centre (4.9749, -12.0104) radius 3.1 projected
  circle A30 centre (-12.0104, -4.9749) radius 3.1 projected
  circle A31 centre (12.0104, -4.9749) radius 3.1 projected
  circle A32 centre (9.1, -76.501) radius 1.6 projected
  circle A33 centre (112.9107, -98.101) radius 1.75 projected
  circle A34 centre (82.8107, -108.101) radius 1.35 projected
  circle A35 centre (58.8107, -108.101) radius 1.35 projected
  circle A36 centre (28.7107, -118.101) radius 1.75 projected
  circle A37 centre (28.7107, -98.101) radius 1.75 projected
  circle A38 centre (70.8107, -120.101) radius 1.35 projected
  circle A39 centre (112.9107, -118.101) radius 1.75 projected
  circle A40 centre (-10.9, -76.501) radius 1.6 projected
  circle A41 centre (58.8107, 108.101) radius 1.35 projected
  circle A42 centre (112.9107, 98.101) radius 1.75 projected
  circle A43 centre (70.8107, 120.101) radius 1.35 projected
  circle A44 centre (28.7107, 118.101) radius 1.75 projected
  circle A45 centre (112.9107, 118.101) radius 1.75 projected
  circle A46 centre (82.8107, 108.101) radius 1.35 projected
  circle A47 centre (28.7107, 98.101) radius 1.75 projected
  line L16 (49.6203, 83.501) -> (49.6203, 93.501) projected
  arc A48 (51.6203, 95.501) -> (49.6203, 93.501) centre (51.6203, 93.501) ccw projected
  line L17 (51.6203, 95.501) -> (90.0011, 95.501) projected
  arc A49 (92.0011, 93.501) -> (90.0011, 95.501) centre (90.0011, 93.501) ccw projected
  line L18 (92.0011, 93.501) -> (92.0011, 83.501) projected
  arc A50 (90.0011, 81.501) -> (92.0011, 83.501) centre (90.0011, 83.501) ccw projected
  line L19 (90.0011, 81.501) -> (51.6203, 81.501) projected
  arc A51 (49.6203, 83.501) -> (51.6203, 81.501) centre (51.6203, 83.501) ccw projected
  circle A52 centre (0, 0) radius 8 projected
  line L20 (15, 93.501) -> (15, 83.501) projected
  arc A53 (13, 81.501) -> (15, 83.501) centre (13, 83.501) ccw projected
  line L21 (13, 81.501) -> (-13, 81.501) projected
  arc A54 (-15, 83.501) -> (-13, 81.501) centre (-13, 83.501) ccw projected
  line L22 (-15, 83.501) -> (-15, 93.501) projected
  arc A55 (-13, 95.501) -> (-15, 93.501) centre (-13, 93.501) ccw projected
  line L23 (-13, 95.501) -> (13, 95.501) projected
  arc A56 (15, 93.501) -> (13, 95.501) centre (13, 93.501) ccw projected
  circle A57 centre (39.1, 76.501) radius 1.6 projected
  circle A58 centre (49.8107, 76.501) radius 1.6 projected
  circle A59 centre (9.1, 76.501) radius 1.6 projected
  circle A60 centre (-10.9, 76.501) radius 1.6 projected
  circle A61 centre (69.8107, 76.501) radius 1.6 projected
  circle A62 centre (89.8107, 76.501) radius 1.6 projected
  circle A63 centre (12.0104, 4.9749) radius 3.1 projected
  circle A64 centre (-4.9749, 12.0104) radius 3.1 projected
  circle A65 centre (-12.0104, 4.9749) radius 3.1 projected
  circle A66 centre (4.9749, 12.0104) radius 3.1 projected
extrude "돌출34" add sketch "스케치30" against normal blind 5 contours A33 | A34 | A35 | A36 | A37 | A38 | A39 | A41 | A42 | A43 | A44 | A45 | A46 | A47
sketch "스케치31" plane through (0, 5, 0) normal (0, 1, 0) x (1, 0, 0)
  circle A0 centre (99.9787, 108.101) radius 1.85 projected
  circle A1 centre (15.7787, -108.101) radius 1.85 projected
  circle A2 centre (35.7787, 108.101) radius 1.75 projected
  circle A3 centre (119.9787, -108.101) radius 1.75 projected
  circle A4 centre (119.9787, 108.101) radius 1.75 projected
  circle A5 centre (35.7787, -108.101) radius 1.75 projected
  circle A6 centre (15.7787, 108.101) radius 1.85 projected
  circle A7 centre (99.9787, -108.101) radius 1.85 projected
  arc A8 (-15.1, 132.9669) -> (-27.1, 120.9669) centre (-15.1, 120.9669) ccw projected
  line L0 (-27.1, 120.9669) -> (-27.1, -120.9669) projected
  arc A9 (-27.1, -120.9669) -> (-15.1, -132.9669) centre (-15.1, -120.9669) ccw projected
  line L1 (-15.1, -132.9669) -> (115.7787, -132.9669) projected
  arc A10 (115.7787, -132.9669) -> (127.7787, -120.9669) centre (115.7787, -120.9669) ccw projected
  line L2 (127.7787, -120.9669) -> (127.7787, -81.2883) projected
  arc A11 (127.7787, -81.2883) -> (120.2094, -70.1362) centre (115.7787, -81.2883) ccw projected
  line L3 (120.2094, -70.1362) -> (34.6692, -36.1508) projected
  arc A12 (27.1, -24.9988) -> (34.6692, -36.1508) centre (39.1, -24.9988) ccw projected
  line L4 (27.1, -24.9988) -> (27.1, 24.9988) projected
  arc A13 (34.6692, 36.1508) -> (27.1, 24.9988) centre (39.1, 24.9988) ccw projected
  line L5 (34.6692, 36.1508) -> (120.2094, 70.1362) projected
  arc A14 (120.2094, 70.1362) -> (127.7787, 81.2883) centre (115.7787, 81.2883) ccw projected
  line L6 (127.7787, 81.2883) -> (127.7787, 120.9669) projected
  arc A15 (127.7787, 120.9669) -> (115.7787, 132.9669) centre (115.7787, 120.9669) ccw projected
  line L7 (115.7787, 132.9669) -> (-15.1, 132.9669) projected
  arc A16 (15, -83.501) -> (13, -81.501) centre (13, -83.501) ccw projected
  line L8 (15, -83.501) -> (15, -93.501) projected
  arc A17 (13, -95.501) -> (15, -93.501) centre (13, -93.501) ccw projected
  line L9 (13, -95.501) -> (-13, -95.501) projected
  arc A18 (-15, -93.501) -> (-13, -95.501) centre (-13, -93.501) ccw projected
  line L10 (-15, -93.501) -> (-15, -83.501) projected
  arc A19 (-13, -81.501) -> (-15, -83.501) centre (-13, -83.501) ccw projected
  line L11 (-13, -81.501) -> (13, -81.501) projected
  line L12 (49.6203, -93.501) -> (49.6203, -83.501) projected
  arc A20 (51.6203, -81.501) -> (49.6203, -83.501) centre (51.6203, -83.501) ccw projected
  line L13 (51.6203, -81.501) -> (90.0011, -81.501) projected
  arc A21 (92.0011, -83.501) -> (90.0011, -81.501) centre (90.0011, -83.501) ccw projected
  line L14 (92.0011, -83.501) -> (92.0011, -93.501) projected
  arc A22 (90.0011, -95.501) -> (92.0011, -93.501) centre (90.0011, -93.501) ccw projected
  line L15 (90.0011, -95.501) -> (51.6203, -95.501) projected
  arc A23 (49.6203, -93.501) -> (51.6203, -95.501) centre (51.6203, -93.501) ccw projected
  circle A24 centre (49.8107, -76.501) radius 1.6 projected
  circle A25 centre (39.1, -76.501) radius 1.6 projected
  circle A26 centre (69.8107, -76.501) radius 1.6 projected
  circle A27 centre (89.8107, -76.501) radius 1.6 projected
  circle A28 centre (-4.9749, -12.0104) radius 3.1 projected
  circle A29 centre (4.9749, -12.0104) radius 3.1 projected
  circle A30 centre (-12.0104, -4.9749) radius 3.1 projected
  circle A31 centre (12.0104, -4.9749) radius 3.1 projected
  circle A32 centre (9.1, -76.501) radius 1.6 projected
  circle A33 centre (-10.9, -76.501) radius 1.6 projected
  line L16 (49.6203, 83.501) -> (49.6203, 93.501) projected
  arc A34 (51.6203, 95.501) -> (49.6203, 93.501) centre (51.6203, 93.501) ccw projected
  line L17 (51.6203, 95.501) -> (90.0011, 95.501) projected
  arc A35 (92.0011, 93.501) -> (90.0011, 95.501) centre (90.0011, 93.501) ccw projected
  line L18 (92.0011, 93.501) -> (92.0011, 83.501) projected
  arc A36 (90.0011, 81.501) -> (92.0011, 83.501) centre (90.0011, 83.501) ccw projected
  line L19 (90.0011, 81.501) -> (51.6203, 81.501) projected
  arc A37 (49.6203, 83.501) -> (51.6203, 81.501) centre (51.6203, 83.501) ccw projected
  circle A38 centre (0, 0) radius 8 projected
  line L20 (15, 93.501) -> (15, 83.501) projected
  arc A39 (13, 81.501) -> (15, 83.501) centre (13, 83.501) ccw projected
  line L21 (13, 81.501) -> (-13, 81.501) projected
  arc A40 (-15, 83.501) -> (-13, 81.501) centre (-13, 83.501) ccw projected
  line L22 (-15, 83.501) -> (-15, 93.501) projected
  arc A41 (-13, 95.501) -> (-15, 93.501) centre (-13, 93.501) ccw projected
  line L23 (-13, 95.501) -> (13, 95.501) projected
  arc A42 (15, 93.501) -> (13, 95.501) centre (13, 93.501) ccw projected
  circle A43 centre (39.1, 76.501) radius 1.6 projected
  circle A44 centre (49.8107, 76.501) radius 1.6 projected
  circle A45 centre (9.1, 76.501) radius 1.6 projected
  circle A46 centre (-10.9, 76.501) radius 1.6 projected
  circle A47 centre (69.8107, 76.501) radius 1.6 projected
  circle A48 centre (89.8107, 76.501) radius 1.6 projected
  circle A49 centre (12.0104, 4.9749) radius 3.1 projected
  circle A50 centre (-4.9749, 12.0104) radius 3.1 projected
  circle A51 centre (-12.0104, 4.9749) radius 3.1 projected
  circle A52 centre (4.9749, 12.0104) radius 3.1 projected
  circle A53 centre (35.7787, -108.101) radius 1.75 projected
  circle A54 centre (99.9787, -108.101) radius 1.85 projected
  line L24 (35.7787, -108.101) -> (99.9787, -108.101) construction
  line L25 (67.8787, -108.101) -> (57.8787, -108.101)
  circle A55 centre (57.8787, -108.101) radius 1.8
  line L26 (67.8787, -108.101) -> (77.8787, -108.101)
  circle A56 centre (77.8787, -108.101) radius 1.8
  dimension "d208" = 10
  dimension "d209" = 3.6
  dimension "d210" = 10
  dimension "d211" = 3.6
  constraints: 6 end point, 2 centre point, 2 coincident, 2 point on line, 1 horizontal, 1 midpoint
  measures "d208" distance of L25.start L25.end
  measures "d209" diameter of A55
  measures "d210" distance of L25.start L26.end
  measures "d211" diameter of A56
extrude "돌출35" cut sketch "스케치31" against normal blind 5 contours A55 | A56
sketch "스케치32" plane through (0, 0, 0) normal (0, 1, 0) x (1, 0, 0)
  circle A0 centre (57.8787, -108.101) radius 1.8 projected
  circle A1 centre (77.8787, -108.101) radius 1.8 projected
  line L0 (57.8787, -108.101) -> (77.8787, -108.101)
  line L1 (47.8787, -118.101) -> (87.8787, -118.101)
  line L2 (87.8787, -118.101) -> (87.8787, -98.101)
  line L3 (87.8787, -98.101) -> (47.8787, -98.101)
  line L4 (47.8787, -98.101) -> (47.8787, -118.101)
  line L5 (47.8787, -118.101) -> (87.8787, -98.101) construction
  line L6 (87.8787, -118.101) -> (47.8787, -98.101) construction
  point P0 (0, 0)
  point P1 (67.8787, -108.101)
  dimension "d214" = 40
  dimension "d215" = 20
  constraints: 14 end point, 3 midpoint, 2 horizontal, 2 parallel, 1 perpendicular
  measures "d214" distance of L3.end L2.end
  measures "d215" distance of L2.end L1.end
extrude "돌출36" cut sketch "스케치32" along normal blind 3
fillet "모깎기7" radius 3 4 edges at (87.8787, 1.5, 98.101) (87.8787, 1.5, 118.101) (47.8787, 1.5, 118.101) (47.8787, 1.5, 98.101)
sketch "스케치33" plane through (0, 0, 0) normal (0, -1, 0) x (1, 0, 0)
  line L0 (50.8787, 118.101) -> (84.8787, 118.101) projected
  arc A0 (87.8787, 115.101) -> (84.8787, 118.101) centre (84.8787, 115.101) ccw projected
  line L1 (87.8787, 115.101) -> (87.8787, 101.101) projected
  arc A1 (84.8787, 98.101) -> (87.8787, 101.101) centre (84.8787, 101.101) ccw projected
  line L2 (84.8787, 98.101) -> (50.8787, 98.101) projected
  arc A2 (47.8787, 101.101) -> (50.8787, 98.101) centre (50.8787, 101.101) ccw projected
  line L3 (47.8787, 101.101) -> (47.8787, 115.101) projected
  arc A3 (50.8787, 118.101) -> (47.8787, 115.101) centre (50.8787, 115.101) ccw projected
  arc A4 (-27.1, -120.9669) -> (-15.1, -132.9669) centre (-15.1, -120.9669) ccw projected
  line L4 (-15.1, -132.9669) -> (115.7787, -132.9669) projected
  arc A5 (115.7787, -132.9669) -> (127.7787, -120.9669) centre (115.7787, -120.9669) ccw projected
  line L5 (127.7787, -120.9669) -> (127.7787, -81.2883) projected
  arc A6 (127.7787, -81.2883) -> (120.2094, -70.1362) centre (115.7787, -81.2883) ccw projected
  line L6 (120.2094, -70.1362) -> (34.6692, -36.1508) projected
  arc A7 (27.1, -24.9988) -> (34.6692, -36.1508) centre (39.1, -24.9988) ccw projected
  line L7 (27.1, 24.9988) -> (27.1, -24.9988) projected
  arc A8 (34.6692, 36.1508) -> (27.1, 24.9988) centre (39.1, 24.9988) ccw projected
  line L8 (34.6692, 36.1508) -> (120.2094, 70.1362) projected
  arc A9 (120.2094, 70.1362) -> (127.7787, 81.2883) centre (115.7787, 81.2883) ccw projected
  line L9 (127.7787, 81.2883) -> (127.7787, 120.9669) projected
  arc A10 (127.7787, 120.9669) -> (115.7787, 132.9669) centre (115.7787, 120.9669) ccw projected
  line L10 (115.7787, 132.9669) -> (-15.1, 132.9669) projected
  arc A11 (-15.1, 132.9669) -> (-27.1, 120.9669) centre (-15.1, 120.9669) ccw projected
  line L11 (-27.1, 120.9669) -> (-27.1, -120.9669) projected
  circle A12 centre (99.9787, -108.101) radius 1.85 projected
  circle A13 centre (15.7787, 108.101) radius 1.85 projected
  circle A14 centre (35.7787, -108.101) radius 1.75 projected
  circle A15 centre (119.9787, 108.101) radius 1.75 projected
  circle A16 centre (119.9787, -108.101) radius 1.75 projected
  circle A17 centre (35.7787, 108.101) radius 1.75 projected
  circle A18 centre (15.7787, -108.101) radius 1.85 projected
  circle A19 centre (99.9787, 108.101) radius 1.85 projected
  circle A20 centre (0, 0) radius 8 projected
  arc A21 (13, 81.501) -> (15, 83.501) centre (13, 83.501) ccw projected
  line L12 (13, 81.501) -> (-13, 81.501) projected
  arc A22 (-15, 83.501) -> (-13, 81.501) centre (-13, 83.501) ccw projected
  line L13 (-15, 83.501) -> (-15, 93.501) projected
  arc A23 (-13, 95.501) -> (-15, 93.501) centre (-13, 93.501) ccw projected
  line L14 (-13, 95.501) -> (13, 95.501) projected
  arc A24 (15, 93.501) -> (13, 95.501) centre (13, 93.501) ccw projected
  line L15 (15, 93.501) -> (15, 83.501) projected
  line L16 (49.6203, 83.501) -> (49.6203, 93.501) projected
  arc A25 (51.6203, 95.501) -> (49.6203, 93.501) centre (51.6203, 93.501) ccw projected
  line L17 (51.6203, 95.501) -> (90.0011, 95.501) projected
  arc A26 (92.0011, 93.501) -> (90.0011, 95.501) centre (90.0011, 93.501) ccw projected
  line L18 (92.0011, 93.501) -> (92.0011, 83.501) projected
  arc A27 (90.0011, 81.501) -> (92.0011, 83.501) centre (90.0011, 83.501) ccw projected
  line L19 (90.0011, 81.501) -> (51.6203, 81.501) projected
  arc A28 (49.6203, 83.501) -> (51.6203, 81.501) centre (51.6203, 83.501) ccw projected
  circle A29 centre (49.8107, 76.501) radius 1.6 projected
  circle A30 centre (39.1, 76.501) radius 1.6 projected
  circle A31 centre (69.8107, 76.501) radius 1.6 projected
  circle A32 centre (89.8107, 76.501) radius 1.6 projected
  circle A33 centre (-4.9749, 12.0104) radius 3.1 projected
  circle A34 centre (4.9749, 12.0104) radius 3.1 projected
  circle A35 centre (-12.0104, 4.9749) radius 3.1 projected
  circle A36 centre (12.0104, 4.9749) radius 3.1 projected
  circle A37 centre (9.1, 76.501) radius 1.6 projected
  circle A38 centre (-10.9, 76.501) radius 1.6 projected
  line L20 (49.6203, -93.501) -> (49.6203, -83.501) projected
  arc A39 (51.6203, -81.501) -> (49.6203, -83.501) centre (51.6203, -83.501) ccw projected
  line L21 (51.6203, -81.501) -> (90.0011, -81.501) projected
  arc A40 (92.0011, -83.501) -> (90.0011, -81.501) centre (90.0011, -83.501) ccw projected
  line L22 (92.0011, -83.501) -> (92.0011, -93.501) projected
  arc A41 (90.0011, -95.501) -> (92.0011, -93.501) centre (90.0011, -93.501) ccw projected
  line L23 (90.0011, -95.501) -> (51.6203, -95.501) projected
  arc A42 (49.6203, -93.501) -> (51.6203, -95.501) centre (51.6203, -93.501) ccw projected
  circle A43 centre (39.1, -76.501) radius 1.6 projected
  circle A44 centre (49.8107, -76.501) radius 1.6 projected
  circle A45 centre (9.1, -76.501) radius 1.6 projected
  circle A46 centre (-10.9, -76.501) radius 1.6 projected
  circle A47 centre (69.8107, -76.501) radius 1.6 projected
  circle A48 centre (89.8107, -76.501) radius 1.6 projected
  circle A49 centre (-12.0104, -4.9749) radius 1.6 projected
  circle A50 centre (4.9749, -12.0104) radius 1.6 projected
  circle A51 centre (12.0104, -4.9749) radius 1.6 projected
  circle A52 centre (-4.9749, -12.0104) radius 1.6 projected
  line L24 (15, -83.501) -> (15, -93.501) projected
  arc A53 (13, -95.501) -> (15, -93.501) centre (13, -93.501) ccw projected
  line L25 (13, -95.501) -> (-13, -95.501) projected
  arc A54 (-15, -93.501) -> (-13, -95.501) centre (-13, -93.501) ccw projected
  line L26 (-15, -93.501) -> (-15, -83.501) projected
  arc A55 (-13, -81.501) -> (-15, -83.501) centre (-13, -83.501) ccw projected
  line L27 (-13, -81.501) -> (13, -81.501) projected
  arc A56 (15, -83.501) -> (13, -81.501) centre (13, -83.501) ccw projected
extrude "돌출37" add sketch "스케치33" against normal blind 5 contours L16 A25 L17 A26 L18 A27 L19 A28 | L20 A39 L21 A40 L22 A41 L23 A42